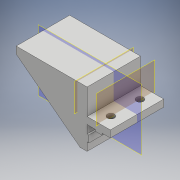
# Autodesk Inventor part: Estrutura - Suporte Z Motor v2
Saved by Autodesk Inventor 2017 (Build 210142000, 142)
## iProperties
Created: 2020-10-04
Part Number: Estrutura - Suporte Z Motor v2
Material: Generic
Document SubType Name: Modeling
Designer: ale
Density: 1 g/cm^3
Appearance: Default
Author: ale
Autodesk Inventor part; units mm, degrees
ref_plane "YZ Plane" through (0, 0, 0) normal (1, 0, 0) x (0, 1, 0)
ref_plane "XZ Plane" through (0, 0, 0) normal (0, 1, 0) x (-1, 0, 0)
ref_plane "XY Plane" through (0, 0, 0) normal (0, 0, 1) x (1, 0, 0)
sketch "Sketch1" plane through (0, 0, 0) normal (0, 0, 1) x (1, 0, 0)
  line L0 (-27.5, 23) -> (27.5, 23)
  line L1 (27.5, 23) -> (27.5, -23)
  line L2 (27.5, -23) -> (-27.5, -23)
  line L3 (-27.5, -23) -> (-27.5, 23)
  line L4 (-27.5, 23) -> (27.5, -23) construction
  line L5 (27.5, 23) -> (-27.5, -23) construction
  point P0 (0, 0)
  dimension "d0" = 55
  dimension "d1" = 46
  constraints: 12 end point, 2 midpoint, 2 parallel, 1 horizontal, 1 perpendicular
  measures "d0" distance of L1.end L2.end
  measures "d1" distance of L0.end L1.end
extrude "Extrusion1" add sketch "Sketch1" along normal blind 6
sketch "Sketch2" plane through (27.5, -23, 0) normal (1, 0, 0) x (0, 0, -1)
  line L0 (-6, 46) -> (-6, 0) projected
  line L1 (-6, 0) -> (16, 0)
  line L2 (16, 0) -> (16, 46)
  line L3 (16, 46) -> (-6, 46)
  line L4 (-6, 46) -> (-6, 0)
  point P0 (0, 23)
  dimension "d4" = 22
  dimension "d5" = 46
  constraints: 8 end point, 2 parallel, 1 horizontal, 1 perpendicular
  measures "d4" distance of L3.end L2.end
  measures "d5" distance of L2.end L1.end
extrude "Extrusion2" add sketch "Sketch2" along normal blind 6
sketch "Sketch4" plane through (27.5, -23, -16) normal (0, 0, -1) x (-1, 0, 0)
  line L0 (0, 0) -> (0, 46) projected
  line L1 (0, 0) -> (-26, 0)
  line L2 (-26, 0) -> (-26, 46)
  line L3 (-26, 46) -> (0, 46)
  line L4 (0, 46) -> (0, 0)
  point P0 (27.5, 23)
  dimension "d8" = 26
  dimension "d35" = 46
  constraints: 8 end point, 2 parallel, 1 horizontal, 1 perpendicular
  measures "d8" distance of L2.end L3.end
  measures "d35" distance between parallel lines of L3 L1
extrude "Extrusion3" add sketch "Sketch4" along normal blind 6
sketch "Sketch5" plane through (27.5, -23, -22) normal (0, 0, -1) x (-1, 0, 0)
  line L0 (0, 46) -> (-26, 46) projected
  line L1 (-6, 0) -> (-26, 0) projected
  line L2 (0, 46) -> (-6, 46)
  line L3 (-6, 46) -> (-6, 0)
  line L4 (-6, 0) -> (0, 0)
  line L5 (0, 0) -> (0, 46)
  point P0 (27.5, 23)
  dimension "d11" = 6
  constraints: 8 end point, 2 parallel, 1 horizontal, 1 perpendicular
  measures "d11" distance of L4.end L1.start
extrude "Extrusion4" add sketch "Sketch5" along normal blind 20
sketch "Sketch6" plane through (27.5, -23, -22) normal (0, 0, -1) x (-1, 0, 0)
  line L0 (-6, 0) -> (-26, 0) projected
  line L1 (-26, 46) -> (-6, 46) projected
  line L2 (-19, 0) -> (-13, 0)
  line L3 (-13, 0) -> (-13, 46)
  line L4 (-13, 46) -> (-19, 46)
  line L5 (-19, 46) -> (-19, 0)
  line L6 (-26, 46) -> (-26, 0) projected
  point P0 (27.5, 23)
  dimension "d14" = 6
  dimension "d15" = 7
  constraints: 8 end point, 2 parallel, 2 point on line, 1 horizontal, 1 perpendicular
  measures "d14" distance of L4.end L3.end
  measures "d15" distance between parallel lines of L6 L5
extrude "Extrusion5" add sketch "Sketch6" along normal blind 1.5 contours L0 L5 L1 L3
sketch "Sketch7" plane through (33.5, -23, -22) normal (1, 0, 0) x (0, 0, -1)
  line L0 (13, 0) -> (7, 0)
  line L1 (7, 0) -> (7, 46)
  line L2 (7, 46) -> (13, 46)
  line L3 (13, 46) -> (13, 0)
  line L4 (20, 46) -> (20, 0) projected
  line L5 (0, 46) -> (20, 46) projected
  point P0 (-22, 23)
  dimension "d18" = 6
  dimension "d19" = 46
  dimension "d20" = 7
  dimension "d36" = 0
  constraints: 8 end point, 2 parallel, 1 horizontal, 1 perpendicular
  measures "d18" distance of L1.end L2.end
  measures "d19" distance of L0.end L1.end
  measures "d20" distance between parallel lines of L4 L3
  measures "d36" distance between parallel lines of L5 L2
extrude "Extrusion6" add sketch "Sketch7" along normal blind 1.5
sketch "Sketch8" plane through (27.5, -23, -23.5) normal (0, 0, -1) x (-1, 0, 0)
  line L0 (-13, 0) -> (-13, 46) projected
  line L1 (-13, 23) -> (-18.895, 23)
  line L2 (-19, 0) -> (-13, 0) projected
  point P0 (27.5, 23)
  point P1 (-16, 10.5)
  point P2 (-16, 35.5)
  dimension "d23" = 10.5
  dimension "d24" = 3
  constraints: 2 end point, 1 horizontal, 1 midpoint, 1 symmetric about line
  measures "d23" distance from line of L2 point (-16, 10.5)
  measures "d24" distance from line of point (-16, 10.5) L0
hole "Hole1" at (43.5, -12.5, -23.5) at (43.5, 12.5, -23.5) direction (0, 0, 1) diameter 6 end through all counterbore diameter 10 counterbore depth 1.5
sketch "Sketch9" plane through (-27.5, -23, 0) normal (0, -1, 0) x (1, 0, 0)
  line L0 (61, -16) -> (61, 6) projected
  line L1 (0, 6) -> (61, 6) projected
  line L2 (61, 6) -> (0, 6)
  line L3 (0, 6) -> (0, 0)
  line L4 (0, 0) -> (54.9849, -42)
  line L5 (55, -42) -> (61, -42) projected
  line L6 (54.9849, -42) -> (61, -42)
  line L7 (61, -42) -> (61, 6)
  point P0 (27.5, 0)
  constraints: 10 end point, 2 perpendicular, 1 horizontal, 1 parallel
extrude "Extrusion7" add sketch "Sketch9" against normal blind 3
ref_plane "Work Plane1" through (-27.5, 0, 6) normal (0, 1, 0) x (1, 0, 0)
mirror "Mirror1" about plane through (-27.5, 0, 6) normal (0, 1, 0) of "Extrusion7"
ref_plane "Work Plane2" through (43.5, -23, 0) normal (1, 0, 0) x (0, 0, -1)
ref_plane "Work Plane3" through (25, -23, 0) normal (1, 0, 0) x (0, 0, -1)
sketch "Sketch11" plane through (27.5, -23, -42) normal (0, 0, -1) x (-1, 0, 0)
  line L0 (0, 3) -> (0, 43) projected
  line L1 (0, 3) -> (-3, 3)
  line L2 (-3, 3) -> (-3, 43)
  line L3 (-3, 43) -> (0, 43)
  line L4 (0, 43) -> (0, 3)
  point P0 (27.5, 23)
  dimension "d39" = 3
  dimension "d40" = 40
  constraints: 8 end point, 2 parallel, 1 horizontal, 1 perpendicular
  measures "d39" distance of L2.end L3.end
  measures "d40" distance of L1.end L2.end
extrude "Extrusion8" cut sketch "Sketch11" against normal blind 42
body "Solid1"
